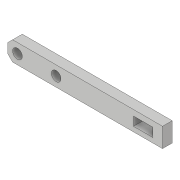
# Autodesk Inventor part: camera_arm
Saved by Autodesk Inventor 2017 (Build 210142000, 142)
## iProperties
Created: 2019-06-13
Part Number: camera_arm
Material: Generic
Document SubType Name: Modeling
Designer: markg
Density: 1 g/cm^3
Appearance: Default
Author: markg
Autodesk Inventor part; units mm, degrees
ref_plane "YZ Plane" through (0, 0, 0) normal (1, 0, 0) x (0, 1, 0)
ref_plane "XZ Plane" through (0, 0, 0) normal (0, 1, 0) x (-1, 0, 0)
ref_plane "XY Plane" through (0, 0, 0) normal (0, 0, 1) x (1, 0, 0)
sketch "Sketch1" plane through (0, 0, 0) normal (0, 0, 1) x (1, 0, 0)
  line L0 (0, 0) -> (50.8, 0)
  line L1 (50.8, 0) -> (50.8, 6.35)
  line L2 (50.8, 6.35) -> (0, 6.35)
  line L3 (0, 6.35) -> (0, 0)
  circle A0 centre (3.175, 3.175) radius 1.5875
  circle A1 centre (15.875, 3.175) radius 1.5875
  line L4 (41.275, 1.5875) -> (47.625, 1.5875)
  line L5 (47.625, 1.5875) -> (47.625, 4.5085)
  line L6 (47.625, 4.5085) -> (41.275, 4.5085)
  line L7 (41.275, 4.5085) -> (41.275, 1.5875)
  dimension "d0" = 50.8
  dimension "d1" = 6.35
  dimension "d2" = 3.175
  dimension "d3" = 3.175
  dimension "d4" = 3.175
  dimension "d5" = 3.175
  dimension "d6" = 3.175
  dimension "d7" = 12.7
  dimension "d8" = 2.921
  dimension "d9" = 1.5875
  dimension "d10" = 6.35
  dimension "d11" = 3.175
  constraints: 16 end point, 4 parallel, 2 centre point, 2 horizontal, 2 perpendicular
  measures "d0" distance of L1.end L2.end
  measures "d1" distance of L0.end L1.end
  measures "d2" distance from line of L0 A0.centre
  measures "d3" distance from line of L0 A1.centre
  measures "d4" diameter of A0
  measures "d5" distance from line of A0.centre L3
  measures "d6" diameter of A1
  measures "d7" distance of A1.centre A0.centre
  measures "d8" distance of L6.end L4.start
  measures "d9" distance between parallel lines of L0 L4
  measures "d10" distance of L4.start L4.end
  measures "d11" distance between parallel lines of L1 L5
extrude "Extrusion1" add sketch "Sketch1" along normal blind 3.175
chamfer "Chamfer1" distance 1.5875 angle 45 2 edges at (0, 6.35, 1.5875) (0, 0, 1.5875)
body "Solid1"
